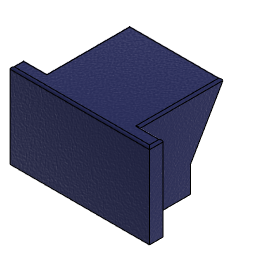
baffle-lock-v2 (Autodesk Fusion 360 design; units mm, degrees)
Autodesk Fusion 360 part; units mm, degrees
sketch "Sketch1" plane through (0, 0, 0) normal (0, 0, 1) x (1, 0, 0)
  line L0 (0, 0) -> (16.5, 0)
  line L1 (16.5, 0) -> (16.5, 1.6)
  line L2 (16.5, 1.6) -> (0, 1.6)
  line L3 (0, 1.6) -> (0, 0)
  line L4 (2.75, 1.6) -> (13.75, 1.6)
  line L5 (13.75, 1.6) -> (13.75, 7.6)
  line L6 (13.75, 7.6) -> (2.75, 7.6)
  line L7 (2.75, 7.6) -> (2.75, 1.6)
  dimension "d1" = 16.5
  dimension "d2" = 1.6
  dimension "d3" = 11
  dimension "d4" = 6
  dimension "d5" = 2.75
  constraint horizontal L0
  constraint vertical L1
  constraint horizontal L2
  constraint vertical L3
  constraint coincident L0.start L3.end
  constraint horizontal L4
  constraint vertical L5
  constraint horizontal L6
  constraint vertical L7
  constraint coincident L2 L4.start
  measures "d1" distance of L0.start L0.end
  measures "d2" distance of L0.start L2.end
  measures "d3" distance of L4.start L4.end
  measures "d4" distance of L4.start L6.end
  measures "d5" distance of L3 L7
extrude "Extrude1" add sketch "Sketch1" along normal blind 10
sketch "Sketch2" plane through (2.75, 0, 0) normal (-1, 0, 0) x (0, -1, 0)
  line L0 (-7.6, 0) -> (-1.6, 0)
  line L1 (-1.6, 0) -> (-1.6, 10)
  line L2 (-1.6, 10) -> (-7.6, 10)
  line L3 (-7.6, 10) -> (-7.6, 0)
  line L4 (-7.6, 10) -> (-11.6, 10)
  line L5 (-11.6, 10) -> (-7.6, 3.0718)
  line L6 (-11.6, 10) -> (-3.6, 10) construction
  dimension "d8" = 4
  dimension "d9" = 60
  constraint coincident L2.end L3.start
  constraint perpendicular L3 L4
  constraint horizontal L6
  constraint coincident L3 L5.end
  measures "d8" distance of L2.end L4.end
  measures "d9" angle of L5 L6
extrude "Extrude2" add sketch "Sketch2" against normal blind 11 contours L3 L4 L5
fillet "Fillet1" radius 0.25 8 edges at (2.75, 6.6, 10) (1.375, 1.6, 10) (0, 0.8, 10) (8.25, 0, 10) (16.5, 0.8, 10) (15.125, 1.6, 10) (13.75, 6.6, 10) (8.25, 11.6, 10)
equation "d5 = ( ( 16.5 - 11 ) / 2 ) * 1 mm"
